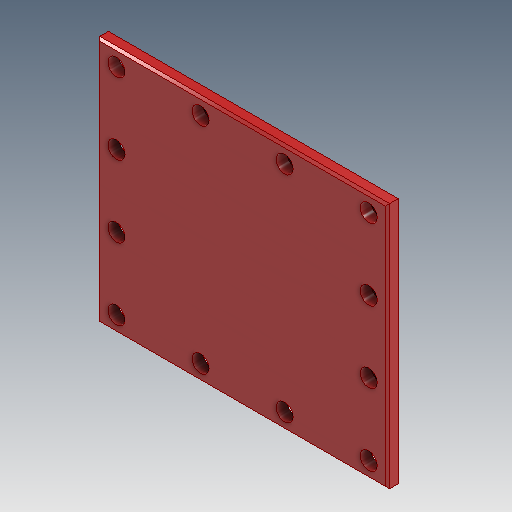
# Autodesk Inventor part: Cover of base
Saved by Autodesk Inventor 2020.3 (Build 243373010, 373A)
## iProperties
Created: 2021-04-25
Part Number: Cover of base
Material: Steel, Alloy
Document SubType Name: Modeling
Designer: marti
Density: 7.73 g/cm^3
Appearance: Red
Mass: 9240.63 g
Surface Area: 1439.94 cm^2
Volume: 1195.42 cm^3
Author: marti
Autodesk Inventor part; units mm, degrees
ref_plane "YZ Plane" through (0, 0, 0) normal (1, 0, 0) x (0, 1, 0)
ref_plane "XZ Plane" through (0, 0, 0) normal (0, 1, 0) x (-1, 0, 0)
ref_plane "XY Plane" through (0, 0, 0) normal (0, 0, 1) x (1, 0, 0)
sketch "Sketch1" plane through (0, 0, 0) normal (0, 0, 1) x (1, 0, 0)
  line L0 (-135, 115) -> (135, 115)
  line L1 (135, 115) -> (135, -115)
  line L2 (135, -115) -> (-135, -115)
  line L3 (-135, -115) -> (-135, 115)
  line L4 (-110, 92.5) -> (110, 92.5)
  line L5 (110, 92.5) -> (110, -92.5)
  line L6 (110, -92.5) -> (-110, -92.5)
  line L7 (-110, -92.5) -> (-110, 92.5)
  point P0 (0, 0)
  point P1 (0, 115)
  point P2 (0, 92.5)
  point P3 (-110, 0)
  point P4 (-135, 0)
  dimension "d0" = 270
  dimension "d1" = 230
  dimension "d2" = 220
  dimension "d3" = 185
  constraints: 16 end point, 4 midpoint, 4 parallel, 2 horizontal, 2 horizontal alignment, 2 perpendicular, 2 vertical alignment
  measures "d0" distance of L1.end L2.end
  measures "d1" distance between parallel lines of L2 L0
  measures "d2" distance between parallel lines of L5 L7
  measures "d3" distance of L6.end L4.start
extrude "Extrusion1" add sketch "Sketch1" against normal blind 15 contours L4 L5 L6 L7
extrude "Extrusion2" add sketch "Sketch1" along normal blind 10 contours L0 L1 L2 L3 | L4 L5 L6 L7
chamfer "Chamfer1" distance 5 angle 45 4 edges at (0, 92.5, -15) (110, 0, -15) (0, -92.5, -15) (-110, 0, -15)
sketch "Sketch2" plane through (0, 0, 10) normal (0, 0, 1) x (1, 0, 0)
  line L0 (125, -107.5) -> (125, 107.5)
  line L1 (-125, 107.5) -> (-125, -107.5)
  line L2 (125, 107.5) -> (-125, 107.5)
  line L3 (-125, -107.5) -> (125, -107.5)
  line L4 (0, 107.5) -> (0, -107.5)
  line L5 (-135, -115) -> (135, -115) projected
  line L6 (135, -115) -> (135, 115) projected
  line L7 (135, 115) -> (-135, 115) projected
  line L8 (-135, 115) -> (-135, -115) projected
  point P0 (0, 0)
  point P1 (-117.5, 100)
  point P2 (-39.1667, 100)
  point P3 (39.1667, 100)
  point P4 (117.5, 100)
  point P5 (-117.5, 33.3333)
  point P6 (-117.5, -33.3333)
  point P7 (-117.5, -100)
  point P8 (-200.4459, 0)
  point P9 (-39.1667, -100)
  point P10 (39.1667, -100)
  point P11 (117.5, -100)
  point P12 (117.5, 33.3333)
  point P13 (117.5, -33.3333)
  dimension "d19" = 250
  dimension "d22" = 7.5
  dimension "d23" = 7.5
  dimension "d24" = 78.3333
  dimension "d25" = 215
  dimension "d26" = 66.6667
  constraints: 10 end point, 2 midpoint, 2 symmetric about line, 1 horizontal, 1 vertical, 9 other
  measures "d19" distance between parallel lines of L0 L1
  measures "d22" distance from line of L2 point (-117.5, 100)
  measures "d23" distance from line of L1 point (-117.5, 100)
  measures "d24" distance of point (-117.5, 100) point (-39.167, 100)
  measures "d25" distance between parallel lines of L3 L2
  measures "d26" distance of point (-117.5, 100) point (-117.5, 33.333)
hole "Hole1" at (117.5, -33.3333, 10) at (117.5, 33.3333, 10) at (117.5, -100, 10) at (39.1667, -100, 10) at (-39.1667, -100, 10) at (-117.5, -100, 10) at (-117.5, -33.3333, 10) at (-117.5, 33.3333, 10) at (117.5, 100, 10) at (39.1667, 100, 10) at (-39.1667, 100, 10) at (-117.5, 100, 10) direction (0, 0, -1) diameter 8.376 depth 27.3 tip angle 118 thread size "M10x1.5" class "6H" standard "ISO Metric profile"
chamfer "Chamfer2" distance 2 angle 45 4 edges at (0, 115, 10) (-135, 0, 10) (135, 0, 10) (0, -115, 10)
sketch "Sketch3" plane through (0, 0, 10) normal (0, 0, 1) x (1, 0, 0)
  circle A0 centre (-117.5, 100) radius 4.188 projected
  circle A1 centre (39.1667, 100) radius 4.188 projected
  circle A2 centre (-117.5, 33.3333) radius 4.188 projected
  circle A3 centre (-117.5, -100) radius 4.188 projected
  circle A4 centre (39.1667, -100) radius 4.188 projected
  circle A5 centre (117.5, 33.3333) radius 4.188 projected
  circle A6 centre (117.5, -33.3333) radius 4.188 projected
  circle A7 centre (117.5, -100) radius 4.188 projected
  circle A8 centre (-39.1667, -100) radius 4.188 projected
  circle A9 centre (-117.5, -33.3333) radius 4.188 projected
  circle A10 centre (117.5, 100) radius 4.188 projected
  circle A11 centre (-39.1667, 100) radius 4.188 projected
  line L0 (133, -113) -> (-133, -113) projected
  line L1 (133, 113) -> (133, -113) projected
  line L2 (-133, 113) -> (133, 113) projected
  line L3 (-133, -113) -> (-133, 113) projected
  circle A12 centre (-117.5, 100) radius 8
  circle A13 centre (-39.167, 100) radius 8
  circle A14 centre (39.166, 100) radius 8
  circle A15 centre (117.499, 100) radius 8
  circle A16 centre (-117.5, 33.333) radius 8
  circle A17 centre (-117.5, -33.334) radius 8
  circle A18 centre (-117.5, -100.001) radius 8
  circle A19 centre (-39.167, -100.001) radius 8
  circle A20 centre (39.166, -100.001) radius 8
  circle A21 centre (117.499, -100.001) radius 8
  circle A22 centre (117.499, 33.333) radius 8
  circle A23 centre (117.499, -33.334) radius 8
  point P0 (0, 0)
  dimension "d39" = 16
  dimension "d42" = 78.333
  dimension "d49" = 66.667
  dimension "d56" = 78.333
  dimension "d63" = 66.667
  constraints: 12 centre point, 2 horizontal, 2 vertical, 1 coincident, 22 other
  measures "d39" diameter of A12
  measures "d42" distance of A12.centre A13.centre
  measures "d49" distance of A12.centre A16.centre
  measures "d56" distance of A18.centre A19.centre
  measures "d63" distance of A15.centre A22.centre
extrude "Extrusion3" cut sketch "Sketch3" against normal blind 10 contours A0 | A1 | A2 | A3 | A4 | A5 | A6 | A7 | A8 | A9 | A10 | A11 | A12 | A13 | A14 | A15 | A16 | A17 | A18 | A19 | A20 | A21 | A22 | A23
equation "\"d22\" = 0.5 * d20"
equation "\"d23\" = 0.5 * d21"
equation "\"d20\" = 15"
equation "\"d21\" = 15"
body "Solid1"
